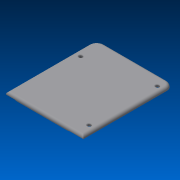
# Autodesk Inventor part: Tampa frente Cartucho MS - 11-05-2016
Saved by Autodesk Inventor 2015 (Build 190159000, 159)
## iProperties
Created: 2016-05-17
Part Number: Tampa frente Cartucho MS - 11-05-2016
Material: Genérico
Document SubType Name: Modeling
Designer: hp
Density: 1 g/cm^3
Appearance: Padrão
Author: hp
Autodesk Inventor part; units mm, degrees
ref_plane "YZ Plane" through (0, 0, 0) normal (1, 0, 0) x (0, 1, 0)
ref_plane "XZ Plane" through (0, 0, 0) normal (0, 1, 0) x (-1, 0, 0)
ref_plane "XY Plane" through (0, 0, 0) normal (0, 0, 1) x (1, 0, 0)
sketch "Esboço1" plane through (0, 0, 0) normal (0, 0, 1) x (1, 0, 0)
  line L0 (-10.4364, 9.1955) -> (73.2016, 9.1955)
  line L1 (73.2016, 9.1955) -> (73.2016, -88.9115)
  line L2 (73.2016, -88.9115) -> (-10.4364, -88.9115)
  line L3 (-10.4364, -88.9115) -> (-10.4364, 9.1955)
  point P0 (0, 0)
  dimension "d0" = 83.638
  dimension "d1" = 98.107
  constraints: 8 end point
  measures "d0" distance of L1.end L2.end
  measures "d1" distance of L0.end L1.end
extrude "Extrusão1" add sketch "Esboço1" along normal blind 3
fillet "Arredondamento1" radius 8 2 edges at (73.2016, 9.1955, 1.5) (-10.4364, 9.1955, 1.5)
sketch "Esboço2" plane through (0, 0, 0) normal (0, 0, -1) x (-1, 0, 0)
  line L0 (-61.1636, -87.6825) -> (6.9824, -87.6825)
  line L1 (6.9824, -87.6825) -> (6.9824, 5.5175)
  line L2 (6.9824, 5.5175) -> (-61.1636, 5.5175)
  line L3 (-61.1636, 5.5175) -> (-61.1636, -87.6825)
  line L4 (2.4364, 9.1955) -> (-65.2016, 9.1955) projected
  line L5 (10.4364, -88.9115) -> (10.4364, 1.1955) projected
  line L6 (-73.2016, -88.9115) -> (10.4364, -88.9115) projected
  point P0 (0, 0)
  dimension "d11" = 68.146
  dimension "d12" = 93.2
  dimension "d14" = 3.454
  dimension "d18" = 1.229
  constraints: 8 end point
  measures "d11" distance of L2.end L1.end
  measures "d12" distance of L1.end L0.end
  measures "d14" distance between parallel lines of L1 L5
  measures "d18" distance between parallel lines of L6 L0
extrude "Extrusão2" add sketch "Esboço2" along normal blind 1.8
fillet "Arredondamento2" radius 7 4 edges at (-6.9824, 5.5175, -0.9) (61.1636, 5.5175, -0.9) (-6.9824, -87.6825, -0.9) (61.1636, -87.6825, -0.9)
sketch "Esboço3" plane through (0, 0, 0) normal (0, 0, -1) x (-1, 0, 0)
  circle A0 centre (-66.3906, -1.7975) radius 1.75
  circle A1 centre (-66.0606, -75.2505) radius 1.75
  circle A2 centre (2.8824, -15.4705) radius 1.75
  line L0 (2.4364, 9.1955) -> (-65.2016, 9.1955) projected
  line L1 (10.4364, -88.9115) -> (10.4364, 1.1955) projected
  line L2 (-73.2016, 1.1955) -> (-73.2016, -88.9115) projected
  line L3 (-73.2016, -88.9115) -> (10.4364, -88.9115) projected
  point P0 (0, 0)
  dimension "d19" = 3.5
  dimension "d20" = 3.5
  dimension "d21" = 3.5
  dimension "d22" = 24.666
  dimension "d23" = 7.554
  dimension "d24" = 6.811
  dimension "d25" = 10.993
  dimension "d26" = 13.661
  dimension "d27" = 7.141
  constraints: 3 centre point
  measures "d19" diameter of A0
  measures "d20" diameter of A1
  measures "d21" diameter of A2
  measures "d22" distance from line of L0 A2.centre
  measures "d23" distance from line of L1 A2.centre
  measures "d24" distance from line of L2 A0.centre
  measures "d25" distance from line of L0 A0.centre
  measures "d26" distance from line of L3 A1.centre
  measures "d27" distance from line of L2 A1.centre
extrude "Extrusão3" cut sketch "Esboço3" against normal blind 4 and the other way blind 4
fillet "Arredondamento3" radius 1 3 edges at (68.1406, -1.7975, 3) (67.8106, -75.2505, 3) (-1.1324, -15.4705, 3)
fillet "Arredondamento4" radius 1 3 edges at (-1.1324, -15.4705, -1.8) (68.1406, -1.7975, 0) (67.8106, -75.2505, 0)
fillet "Arredondamento5" radius 3 6 edges at (-10.4364, -43.858, 3) (-8.0933, 6.8523, 3) (31.3826, 9.1955, 3) (70.8584, 6.8523, 3) (73.2016, -43.858, 3) (31.3826, -88.9115, 3)
